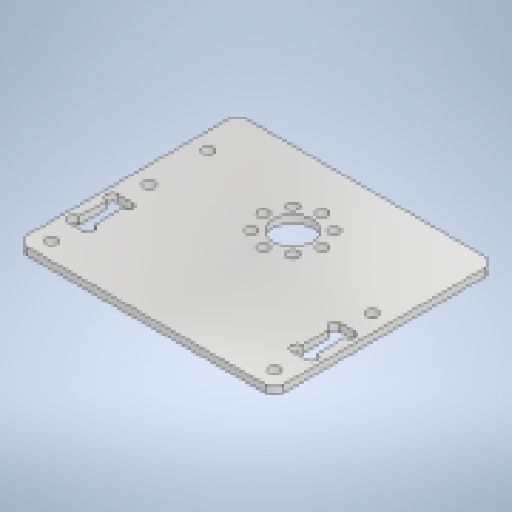
# Autodesk Inventor part: kosi_v3_1.5
Saved by Autodesk Inventor 2025.1 (Build 291241000, 241)
## iProperties
Created: 2024-09-01
Part Number: kosi_v3_1.5
Material: アルミニウム 2014-T4
Document SubType Name: Modeling
Designer: right
Density: 2.8 g/cm^3
Appearance: サテン
Mass: 9.17355 g
Surface Area: 49.2125 cm^2
Volume: 3.27627 cm^3
Author: right
Autodesk Inventor part; units mm, degrees
ref_plane "YZ Plane" through (0, 0, 0) normal (1, 0, 0) x (0, 1, 0)
ref_plane "XZ Plane" through (0, 0, 0) normal (0, 1, 0) x (-1, 0, 0)
ref_plane "XY Plane" through (0, 0, 0) normal (0, 0, 1) x (1, 0, 0)
sketch "スケッチ1" plane through (0, 0, 0) normal (0, 1, 0) x (-1, 0, 0)
  circle A0 centre (0, 0) radius 4
  circle A1 centre (0, 0) radius 8
  circle A2 centre (0, 0) radius 6 construction
  circle A3 centre (0, -6) radius 1.1
  circle A4 centre (4.2426, -4.2426) radius 1.1
  circle A5 centre (6, 0) radius 1.1
  circle A6 centre (4.2426, 4.2426) radius 1.1
  circle A7 centre (0, 6) radius 1.1
  circle A8 centre (-4.2426, 4.2426) radius 1.1
  circle A9 centre (-6, 0) radius 1.1
  circle A10 centre (-4.2426, -4.2426) radius 1.1
  line L0 (26.25, -15) -> (-26.25, -15)
  line L1 (-26.25, -15) -> (-26.25, 30)
  line L2 (-26.25, 30) -> (26.25, 30)
  line L3 (26.25, 30) -> (26.25, -15)
  line L4 (24.25, 11.5) -> (21.25, 11.5)
  line L5 (21.25, 11.5) -> (21.25, 21.5)
  line L6 (21.25, 21.5) -> (24.25, 21.5)
  line L7 (24.25, 21.5) -> (24.25, 11.5)
  circle A11 centre (24.25, 12.6) radius 1.1
  circle A12 centre (21.25, 12.6) radius 1.1
  line L8 (0, 0) -> (0, -15) construction
  circle A13 centre (24.25, 20.4) radius 1.1
  circle A14 centre (21.25, 20.4) radius 1.1
  line L9 (-24.25, 11.5) -> (-21.25, 11.5)
  line L10 (-21.25, 11.5) -> (-21.25, 21.5)
  line L11 (-21.25, 21.5) -> (-24.25, 21.5)
  line L12 (-24.25, 21.5) -> (-24.25, 11.5)
  circle A15 centre (-24.25, 12.6) radius 1.1
  circle A16 centre (-21.25, 12.6) radius 1.1
  circle A17 centre (-24.25, 20.4) radius 1.1
  circle A18 centre (-21.25, 20.4) radius 1.1
  circle A19 centre (22.75, 6.5) radius 1.1
  circle A20 centre (22.75, 26.5) radius 1.1
  circle A21 centre (-22.75, 6.5) radius 1.1
  circle A22 centre (-22.75, 26.5) radius 1.1
  circle A23 centre (22.75, 26.5) radius 3.5 construction
  point P0 (21.25, 16.5)
  point P1 (-21.25, 16.5)
  point P2 (22.75, 11.5)
  point P3 (-21.25, 19.3)
  point P4 (-21.25, 13.7)
  point P5 (-24.25, 13.7)
  point P6 (-24.25, 19.3)
  point P7 (-24.25, 21.5)
  point P8 (-21.25, 21.5)
  point P9 (21.25, 19.3)
  point P10 (21.25, 21.5)
  point P11 (24.25, 21.5)
  point P12 (24.25, 19.3)
  point P13 (24.25, 13.7)
  point P14 (21.25, 13.7)
  point P15 (22.75, 21.5)
  dimension "d2" = 12
  dimension "d10" = 2.2
  dimension "d0" = 8
  dimension "d1" = 16
  dimension "d3" = 2.2
  dimension "d6" = 360
  dimension "d8" = 3
  dimension "d9" = 10
  dimension "d11" = 42.5
  dimension "d12" = 2.2
  dimension "d13" = 5
  dimension "d17" = 5
  dimension "d18" = 7
  dimension "d29" = 45
  dimension "d30" = 30
  constraints: 26 end point, 19 centre point, 11 symmetric about line, 6 point on line, 5 vertical alignment, 4 coincident, 4 midpoint, 4 parallel, 4 tangent, 2 equal radius, 2 horizontal, 2 perpendicular, 2 vertical, 36 other
  measures "d0" diameter of A0
  measures "d1" diameter of A1
  measures "d3" diameter of A3
  measures "d8" distance of L4.start L4.end
  measures "d9" distance of L4.end L5.end
  measures "d11" distance between parallel lines of L10 L5
  measures "d12" diameter of A19
  measures "d13" distance from line of L4 A19.centre
  measures "d17" distance of point (22.75, 21.5) A20.centre
  measures "d18" diameter of A23
  measures "d29" distance of L0.end L1.end
  measures "d30" distance from line of L2 point (0, 0)
extrude "押し出し1" add sketch "スケッチ1" along normal blind 1.5 contours A1 | L0 L1 L2 L3
sketch "スケッチ2" plane through (0, 0, 0) normal (0, -1, 0) x (1, 0, 0)
  circle A0 centre (-22.75, -5.5) radius 1.1
  circle A1 centre (-22.75, 6.5) radius 1.1 projected
  point P0 (0, 0)
  dimension "d19" = 2.2
  dimension "d20" = 12
  constraints: 1 centre point, 1 vertical alignment
  measures "d19" diameter of A0
  measures "d20" distance of A0.centre A1.centre
extrude "押し出し2" cut sketch "スケッチ2" against normal through all contours A0
fillet "フィレット1" radius 2 4 edges at (-26.25, 0.75, -15) (26.25, 0.75, -15) (26.25, 0.75, 30) (-26.25, 0.75, 30)
equation "\"d17\" = d13"
